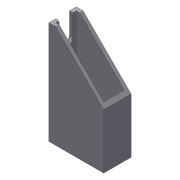
# Autodesk Inventor part: FrameSideBumperMounts
Saved by Autodesk Inventor 2012 (Build 160160000, 160)
## iProperties
Created: 2013-01-07
Part Number: FrameSideBumperMounts
Material: Aluminum-6061
Document SubType Name: Modeling
Designer: JesseK
Mass: 87.8378 g
Surface Area: 215.789 cm^2
Volume: 32.4125 cm^3
Density: 2.71 g/cm^3
Author: JesseK
Autodesk Inventor part; units mm, degrees
ref_plane "YZ Plane" through (0, 0, 0) normal (1, 0, 0) x (0, 1, 0)
ref_plane "XZ Plane" through (0, 0, 0) normal (0, 1, 0) x (-1, 0, 0)
ref_plane "XY Plane" through (0, 0, 0) normal (0, 0, 1) x (1, 0, 0)
sketch "Sketch1" plane through (0, 0, 0) normal (0, 0, 1) x (1, 0, 0)
  line L0 (0, 0) -> (50.8, 0)
  line L1 (50.8, 0) -> (50.8, 101.6)
  line L2 (50.8, 101.6) -> (0, 101.6)
  line L3 (0, 101.6) -> (0, 0)
  dimension "d3" = 50.8
  dimension "d4" = 101.6
  constraints: 8 end point, 2 parallel, 1 horizontal, 1 perpendicular
  measures "d3" distance of L1.end L2.end
  measures "d4" distance of L2.end L0.start
extrude "Extrusion1" add sketch "Sketch1" along normal blind 25.4
shell "Shell1" thickness 3.175 removed faces 2 at (33.8667, 101.6, 16.9333) at (16.9333, 0, 16.9333)
sketch "Sketch2" plane through (0, 0, 0) normal (0, 0, -1) x (-1, 0, 0)
  line L0 (-50.8, 101.6) -> (0, 101.6) projected
  line L1 (-50.8, 0) -> (-50.8, 101.6) projected
  line L2 (-50.8, 50.8) -> (-50.8, 101.6)
  line L3 (-50.8, 101.6) -> (0, 101.6)
  line L4 (0, 101.6) -> (-50.8, 50.8)
  dimension "d5" = 50.8
  constraints: 6 end point, 1 horizontal, 1 midpoint, 1 vertical
  measures "d5" distance of L2.start L0.start
extrude "Extrusion2" cut sketch "Sketch2" against normal through all
sketch "Sketch3" plane through (0, 0, 0) normal (-1, 0, 0) x (0, 0, 1)
  line L0 (0, 101.6) -> (25.4, 101.6) projected
  line L1 (0, 101.6) -> (0, 0) projected
  arc A0 (6.35, 76.2) -> (19.05, 76.2) centre (12.7, 76.2) ccw
  line L2 (6.35, 76.2) -> (6.35, 101.6)
  line L3 (19.05, 76.2) -> (19.05, 101.6)
  dimension "d8" = 25.4
  dimension "d9" = 6.35
  dimension "d10" = 12.7
  constraints: 4 end point, 2 point on circle, 2 point on line, 2 tangent, 2 vertical, 1 centre point
  measures "d8" distance of L3.start L3.end
  measures "d9" radius of A0
  measures "d10" distance from line of L1 A0.centre
extrude "Extrusion3" cut sketch "Sketch3" against normal through all
chamfer "Chamfer1" distance 3.175 angle 45 2 edges at (1.5875, 100.0125, 6.35) (1.5875, 100.0125, 19.05)
sketch "Sketch4" plane through (0, 0, 25.4) normal (0, 0, 1) x (1, 0, 0)
  line L0 (50.8, 50.8) -> (0, 101.6) projected
  line L1 (0, 0) -> (0, 101.6) projected
  line L2 (0, 101.6) -> (0, 95.25)
  line L3 (6.35, 95.25) -> (0, 101.6)
  line L4 (0, 95.25) -> (6.35, 95.25)
  dimension "d16" = 6.35
  constraints: 6 end point, 2 point on line, 1 collinear, 1 horizontal
  measures "d16" distance of L0.end L2.end
extrude "Extrusion4" cut sketch "Sketch4" against normal through all
body "Solid1"
